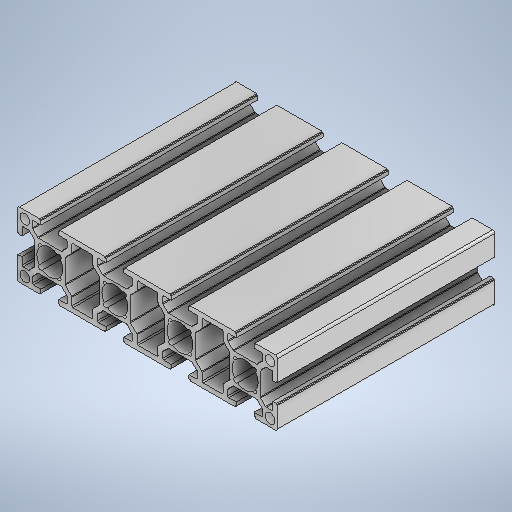
# Autodesk Inventor part: Sessao_04_04
Saved by Autodesk Inventor 2026 (Build 300175000, 175)
## iProperties
Created: 2025-04-04
Part Number: Sessao_04_04
Material: Aluminum 6061
Document SubType Name: Modeling
Designer: Carlos Dias
Density: 2.7 g/cm^3
Appearance: Aluminum - Polished
Author: Carlos Dias
Autodesk Inventor part; units mm, degrees
sketch "Sketch1" plane through (0, 0, 0) normal (0, 0, 1) x (1, 0, 0)
  line L0 (-60, 15) -> (-60, 0) construction
  line L1 (-60, 15) -> (-60, 4.1) construction
  line L2 (-60, 4.1) -> (-57.8, 4.1) construction
  line L3 (-57.8, 8) -> (-57.8, 4.1) construction
  line L4 (-60, 4.1) -> (-59.5, 4.1) construction
  line L5 (-59.5, 4.1) -> (-59.5, 4.6)
  line L6 (-59.5, 4.6) -> (-60, 4.6)
  line L7 (-60, 4.6) -> (-60, 4.1) construction
  line L8 (-60, 15) -> (-60, 4.6) construction
  line L9 (-57.8, 4.1) -> (-59.5, 4.1)
  line L10 (-60, 15) -> (0, 15) construction
  arc A0 (-59, 15) -> (-60, 14) centre (-59, 14) ccw
  line L11 (-60, 14) -> (-60, 4.6)
  circle A1 centre (-56.5, 11.5) radius 2.25
  circle A2 centre (-45, 0) radius 6 construction
  line L12 (-49.1, 15) -> (-49.1, 12.8) construction
  line L13 (-49.1, 15) -> (-49.6, 15) construction
  line L14 (-49.6, 15) -> (-49.6, 14.5)
  line L15 (-49.6, 14.5) -> (-49.1, 14.5)
  line L16 (-49.1, 14.5) -> (-49.1, 15) construction
  line L17 (-49.1, 14.5) -> (-49.1, 12.8)
  line L18 (-59, 15) -> (-49.6, 15)
  line L19 (-53, 12.8) -> (-49.1, 12.8) construction
  line L20 (-57.8, 8) -> (-52, 8) construction
  arc A3 (-57.3, 8) -> (-57.8, 7.5) centre (-57.3, 7.5) ccw
  line L21 (-57.8, 7.5) -> (-57.8, 4.1)
  line L22 (-52, 5.4444) -> (-52, 0) construction
  line L23 (-60, 15) -> (-45, 0) construction
  circle A4 centre (-49.2426, 4.2426) radius 1 construction
  circle A5 centre (-45, 0) radius 6 construction
  circle A6 centre (-49.2426, -4.2426) radius 1 construction
  circle A7 centre (-45, 0) radius 6 construction
  circle A8 centre (-40.7574, -4.2426) radius 1 construction
  circle A9 centre (-45, 0) radius 6 construction
  circle A10 centre (-40.7574, 4.2426) radius 1 construction
  line L24 (-50.4444, 7) -> (-45, 7) construction
  line L25 (-53, 9.5556) -> (-50.4444, 7) construction
  line L26 (-54.5556, 8) -> (-52, 5.4444) construction
  line L27 (-53, 12.8) -> (-53, 9.5556) construction
  line L28 (-45, 7) -> (-39.5556, 7) construction
  line L29 (-40.9, 12.8) -> (-37, 12.8) construction
  line L30 (-40.9, 15) -> (-40.9, 12.8) construction
  line L31 (-40.9, 15) -> (-40.4, 15) construction
  line L32 (-40.4, 15) -> (-40.4, 14.5)
  line L33 (-40.4, 14.5) -> (-40.9, 14.5)
  line L34 (-40.9, 14.5) -> (-40.9, 15) construction
  line L35 (-40.9, 14.5) -> (-40.9, 12.8)
  line L36 (-37, 12.8) -> (-37, 9.5556) construction
  line L37 (-37, 9.5556) -> (-39.5556, 7) construction
  line L38 (-15, 15) -> (-19.1, 15) construction
  line L39 (-38, 5.4444) -> (-38, 0) construction
  line L40 (-34.8, 8.6444) -> (-38, 5.4444) construction
  line L41 (-34.8, 12.8) -> (-34.8, 8.6444) construction
  circle A11 centre (-15, 0) radius 6 construction
  line L42 (-34.8, 12.8) -> (-25.2, 12.8) construction
  line L43 (-30, 15) -> (-15, 0) construction
  circle A12 centre (-19.2426, 4.2426) radius 1 construction
  circle A13 centre (-19.2426, -4.2426) radius 1 construction
  circle A14 centre (-10.7574, -4.2426) radius 1 construction
  circle A15 centre (-10.7574, 4.2426) radius 1 construction
  line L44 (-20.4444, 7) -> (-9.5556, 7) construction
  line L45 (-22, 5.4444) -> (-22, 0) construction
  line L46 (-23, 9.5556) -> (-20.4444, 7) construction
  line L47 (-25.2, 8.6444) -> (-22, 5.4444) construction
  line L48 (-25.2, 12.8) -> (-25.2, 8.6444) construction
  line L49 (-23, 12.8) -> (-23, 9.5556) construction
  line L50 (-19.1, 15) -> (-19.1, 12.8) construction
  line L51 (-19.1, 12.8) -> (-23, 12.8) construction
  line L52 (-19.1, 15) -> (-19.6, 15) construction
  line L53 (-19.6, 15) -> (-19.6, 14.5)
  line L54 (-19.6, 14.5) -> (-19.1, 14.5)
  line L55 (-19.1, 14.5) -> (-19.1, 15) construction
  line L56 (-19.1, 14.5) -> (-19.1, 12.8)
  line L57 (-40.4, 15) -> (-19.6, 15)
  arc A16 (-49.8884, 3.4791) -> (-51, 0) centre (-45, 0) ccw
  arc A17 (-41.5209, 4.8884) -> (-48.4791, 4.8884) centre (-45, 0) ccw
  arc A18 (-39, 0) -> (-40.1116, 3.4791) centre (-45, 0) ccw
  arc A19 (-48.4791, 4.8884) -> (-49.8884, 3.4791) centre (-49.2426, 4.2426) ccw
  arc A20 (-40.1116, 3.4791) -> (-41.5209, 4.8884) centre (-40.7574, 4.2426) ccw
  line L58 (-72.2485, 0) -> (12.0414, 0) projected
  line L59 (-8, 5.4444) -> (-8, 0) construction
  line L60 (0, 15) -> (-15, 0) construction
  line L61 (-7, 9.5556) -> (-9.5556, 7) construction
  line L62 (-4.8, 8.6444) -> (-8, 5.4444) construction
  arc A21 (-19.8884, 3.4791) -> (-21, 0) centre (-15, 0) ccw
  arc A22 (-18.4791, 4.8884) -> (-19.8884, 3.4791) centre (-19.2426, 4.2426) ccw
  arc A23 (-11.5209, 4.8884) -> (-18.4791, 4.8884) centre (-15, 0) ccw
  arc A24 (-10.1116, 3.4791) -> (-11.5209, 4.8884) centre (-10.7574, 4.2426) ccw
  arc A25 (-9, 0) -> (-10.1116, 3.4791) centre (-15, 0) ccw
  line L63 (-7, 12.8) -> (-7, 9.5556) construction
  line L64 (-4.8, 12.8) -> (-4.8, 8.6444) construction
  line L65 (-10.9, 12.8) -> (-7, 12.8) construction
  line L66 (-10.9, 12.8) -> (-10.9, 15) construction
  line L67 (-4.8, 12.8) -> (-0.5, 12.8) construction
  line L68 (-10.9, 15) -> (-10.4, 15) construction
  line L69 (-10.4, 15) -> (-10.4, 14.5)
  line L70 (-10.4, 14.5) -> (-10.9, 14.5)
  line L71 (-10.9, 14.5) -> (-10.9, 15) construction
  line L72 (-10.9, 14.5) -> (-10.9, 12.8)
  line L73 (-10.4, 15) -> (0, 15)
  line L74 (0, 19.4485) -> (0, -10.2414) projected
  arc A26 (-54.4092, 7.8536) -> (-54.7627, 8) centre (-54.7627, 7.5) ccw
  arc A27 (-52, 5.2373) -> (-52.1464, 5.5908) centre (-52.5, 5.2373) ccw
  line L75 (-57.3, 8) -> (-54.7627, 8)
  line L76 (-54.4092, 7.8536) -> (-52.1464, 5.5908)
  line L77 (-52, 5.2373) -> (-52, 0)
  line L78 (-52, 0) -> (-51, 0)
  arc A28 (-53, 9.7627) -> (-52.8536, 9.4092) centre (-52.5, 9.7627) ccw
  arc A29 (-50.5908, 7.1464) -> (-50.2373, 7) centre (-50.2373, 7.5) ccw
  arc A30 (-52.5, 12.8) -> (-53, 12.3) centre (-52.5, 12.3) ccw
  arc A31 (-37, 12.3) -> (-37.5, 12.8) centre (-37.5, 12.3) ccw
  arc A32 (-37.1464, 9.4092) -> (-37, 9.7627) centre (-37.5, 9.7627) ccw
  arc A33 (-39.7627, 7) -> (-39.4092, 7.1464) centre (-39.7627, 7.5) ccw
  arc A34 (-37.8536, 5.5908) -> (-38, 5.2373) centre (-37.5, 5.2373) ccw
  arc A35 (-34.9464, 8.4979) -> (-34.8, 8.8515) centre (-35.3, 8.8515) ccw
  arc A36 (-34.3, 12.8) -> (-34.8, 12.3) centre (-34.3, 12.3) ccw
  arc A37 (-25.2, 12.3) -> (-25.7, 12.8) centre (-25.7, 12.3) ccw
  arc A38 (-25.2, 8.8515) -> (-25.0536, 8.4979) centre (-24.7, 8.8515) ccw
  arc A39 (-22, 5.2373) -> (-22.1464, 5.5908) centre (-22.5, 5.2373) ccw
  line L79 (-38, 5.2373) -> (-38, 0)
  line L80 (-38, 0) -> (-39, 0)
  line L81 (-34.9464, 8.4979) -> (-37.8536, 5.5908)
  line L82 (-34.8, 12.3) -> (-34.8, 8.8515)
  line L83 (-52.5, 12.8) -> (-49.1, 12.8)
  line L84 (-53, 12.3) -> (-53, 9.7627)
  line L85 (-52.8536, 9.4092) -> (-50.5908, 7.1464)
  line L86 (-50.2373, 7) -> (-39.7627, 7)
  line L87 (-37.1464, 9.4092) -> (-39.4092, 7.1464)
  line L88 (-37, 12.3) -> (-37, 9.7627)
  line L89 (-40.9, 12.8) -> (-37.5, 12.8)
  line L90 (-34.3, 12.8) -> (-25.7, 12.8)
  line L91 (-25.2, 12.3) -> (-25.2, 8.8515)
  line L92 (-25.0536, 8.4979) -> (-22.1464, 5.5908)
  line L93 (-22, 5.2373) -> (-22, 0)
  line L94 (-22, 0) -> (-21, 0)
  arc A40 (-22.5, 12.8) -> (-23, 12.3) centre (-22.5, 12.3) ccw
  arc A41 (-23, 9.7627) -> (-22.8536, 9.4092) centre (-22.5, 9.7627) ccw
  arc A42 (-20.5908, 7.1464) -> (-20.2373, 7) centre (-20.2373, 7.5) ccw
  arc A43 (-9.7627, 7) -> (-9.4092, 7.1464) centre (-9.7627, 7.5) ccw
  arc A44 (-7.1464, 9.4092) -> (-7, 9.7627) centre (-7.5, 9.7627) ccw
  arc A45 (-7, 12.3) -> (-7.5, 12.8) centre (-7.5, 12.3) ccw
  arc A46 (-4.9464, 8.4979) -> (-4.8, 8.8515) centre (-5.3, 8.8515) ccw
  arc A47 (-7.8536, 5.5908) -> (-8, 5.2373) centre (-7.5, 5.2373) ccw
  arc A48 (-4.3, 12.8) -> (-4.8, 12.3) centre (-4.3, 12.3) ccw
  line L95 (-22.5, 12.8) -> (-19.1, 12.8)
  line L96 (-23, 12.3) -> (-23, 9.7627)
  line L97 (-22.8536, 9.4092) -> (-20.5908, 7.1464)
  line L98 (-20.2373, 7) -> (-9.7627, 7)
  line L99 (-7.1464, 9.4092) -> (-9.4092, 7.1464)
  line L100 (-7, 12.3) -> (-7, 9.7627)
  line L101 (-10.9, 12.8) -> (-7.5, 12.8)
  line L102 (-8, 5.2373) -> (-8, 0)
  line L103 (-8, 0) -> (-8, 5.2373)
  line L104 (-9, 0) -> (-8, 0)
  line L105 (-4.9464, 8.4979) -> (-7.8536, 5.5908)
  line L106 (-4.8, 12.3) -> (-4.8, 8.8515)
  line L107 (-4.3, 12.8) -> (0, 12.8)
  line L108 (0, 12.8) -> (0, 15)
  point P0 (0, 0)
  point P1 (-22.5, 7.5)
  dimension "d33" = 12
  dimension "d0" = 60
  dimension "d2" = 15
  dimension "d3" = 4.1
  dimension "d4" = 2.2
  dimension "d6" = 0.5
  dimension "d7" = 1
  dimension "d8" = 4.5
  dimension "d32" = 45
  dimension "d34" = 4.1
  dimension "d37" = 56.5
  dimension "d38" = 11.5
  dimension "d39" = 1.25
  dimension "d40" = 0.5
  dimension "d42" = 8
  dimension "d46" = 2
  dimension "d49" = 360
  dimension "d51" = 1
  dimension "d52" = 1.1
  dimension "d54" = 8.2
  dimension "d55" = 15
  dimension "d56" = 2.2
  dimension "d57" = 1
  dimension "d58" = 2.2
  dimension "d62" = 360
  dimension "d64" = 1
  dimension "d65" = 1
  dimension "d66" = 1.1
  dimension "d69" = 21.3
  dimension "d70" = 1
  dimension "d71" = 1.1
  constraints: 216 end point, 78 point on circle, 57 point on line, 50 tangent, 44 centre point, 33 vertical, 31 horizontal, 24 equal radius, 19 equal length, 17 parallel, 16 coincident, 14 horizontal alignment, 5 perpendicular, 4 concentric, 3 vertical alignment, 2 midpoint, 1 collinear, 70 other
  measures "d0" horizontal distance of L0.start point (0, 0)
  measures "d2" distance of L0.start L0.end
  measures "d3" vertical distance of point (0, 0) L1.end
  measures "d4" distance of L1.end L2.end
  measures "d6" distance of L5.end L6.end
  measures "d7" radius of A0
  measures "d8" diameter of A1
  measures "d32" distance of point (0, 0) point (-45, 0)
  measures "d34" horizontal distance of L12.start point (-45, 0)
  measures "d37" horizontal distance of point (0, 0) A1.centre
  measures "d38" vertical distance of point (0, 0) A1.centre
  measures "d39" distance edge to line of A1 L20
  measures "d40" radius of A3
  measures "d42" horizontal distance of L1.end L22.end
  measures "d46" diameter of A4
  measures "d52" distance between parallel lines of L23 L25
  measures "d54" distance of L29.start L12.end
  measures "d55" horizontal distance of point (0, 0) L38.start
  measures "d56" distance of L29.end L41.start
  measures "d58" distance between parallel lines of L37 L40
  measures "d66" distance between parallel lines of L43 L46
  measures "d69" distance of L31.end L38.end
  measures "d71" distance between parallel lines of L60 L61
extrude "Extrusion1" add sketch "Sketch1" along normal mid plane 100 contours L5 L6 L11 A0 L18 L14 L15 L17 L83 A30 L84 A28 L85 A29 L86 A33 L87 A32 L88 A31 L89 L35 L33 L32 L57 L53 L54 L56 L95 A40 L96 A41 L97 A42 L98 A43 L99 A44 L100 A45 L101 L72 L70 L69 L73 L74 L107 A48 L106 A46 L105 A47 L102 L58 A25 A24 A23 A22 A21 L93 A39 L92 A38 L91 A37 L90 A36 L82 A35 L81 A34 L79 A18 A20 A17 A19 A16 L77 A27 L76 A26 L75 A3 L21 L9
mirror "Mirror1" about plane through (0, 0, 0) normal (0, 1, 0) of "Extrusion1"
mirror "Mirror2" about plane through (0, 0, 0) normal (1, 0, 0) of "Extrusion1", "Mirror1"
equation "\"d52\" = 0.5 * d4"
equation "\"d56\" = d4"
equation "\"d57\" = d51"
equation "\"d58\" = d4"
body "Solid1"
